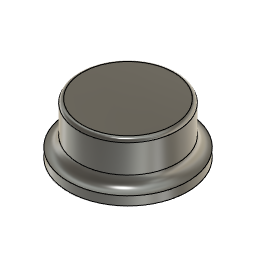
Knob_V1 (Autodesk Fusion 360 design; units mm, degrees)
Autodesk Fusion 360 part; units mm, degrees
sketch "Sketch1" plane through (0, 0, 0) normal (0, 0, 1) x (1, 0, 0)
  line L0 (-1.45, 2.6263) -> (-1.45, -2.6263) construction
  arc A0 (-1.45, -2.6263) -> (-1.45, 2.6263) centre (0, 0) ccw construction
  arc A1 (-1.63, -2.7305) -> (-1.63, 2.7305) centre (0, 0) ccw
  line L1 (-1.63, 2.7305) -> (-1.63, -2.7305)
  circle A2 centre (0, 0) radius 17
  circle A3 centre (0, 0) radius 14
  dimension "d1" = 6
  dimension "d4" = 0.18
  dimension "d5" = 34
  dimension "d6" = 3
  constraint coincident A0.centre A1.centre
  constraint vertical L0
  constraint concentric A0 A3
  measures "d1" diameter of A0
  measures "d5" diameter of A2
  measures "d6" distance of A2 A3
extrude "Extrude1" add sketch "Sketch1" along normal blind 14 contours A1 L1 | A3
extrude "Extrude2" add sketch "Sketch1" along normal blind 2 contours A2
extrude "Extrude3" cut sketch "Sketch1" along normal blind 12 contours A1 L1
fillet "Fillet1" radius 3 1 edges at (-13.0526, -5.0626, 2)
fillet "Fillet2" radius 1 1 edges at (-13.0526, -5.0626, 14)
extrude "Extrude4" add sketch "Sketch1" along normal blind 2 contours A2
extrude "Extrude5" add sketch "Sketch1" against normal blind 0.5 contours A2 | A3
equation "mountTol = 0.18 mm"
equation "d4 = mountTol"
